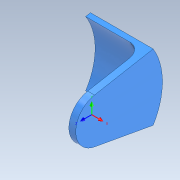
# Autodesk Inventor part: thigh_connector
Saved by Autodesk Inventor 2020 (Build 240168000, 168)
## iProperties
Created: 2021-03-27
Part Number: thigh_connector
Material: Generic
Document SubType Name: Modeling
Designer: DELL
Density: 1 g/cm^3
Appearance: Cyan
Author: DELL
Autodesk Inventor part; units mm, degrees
ref_plane "YZ Plane" through (0, 0, 0) normal (1, 0, 0) x (0, 1, 0)
ref_plane "XZ Plane" through (0, 0, 0) normal (0, 1, 0) x (-1, 0, 0)
ref_plane "XY Plane" through (0, 0, 0) normal (0, 0, 1) x (1, 0, 0)
sketch "Sketch1" plane through (0, 0, 0) normal (1, 0, 0) x (0, 1, 0)
  circle A0 centre (0, 0) radius 20
  line L0 (-19.68, 3.5636) -> (-29, -47.9062)
  line L1 (19.68, 3.5636) -> (29, -47.9062)
  line L2 (11.5, 0) -> (-11.5, 0) construction
  line L3 (0, -48.5721) -> (0, 48.5721) construction
  arc A1 (-28.2326, -43.6683) -> (28.2326, -43.6683) centre (0, 0) ccw
  arc A2 (-29, -47.9062) -> (29, -47.9062) centre (0, 0) ccw
  point P0 (0, -56)
  point P1 (0, 0)
  dimension "d0" = 40
  dimension "d8" = 104
  dimension "d9" = 112
  dimension "d10" = 58
  constraints: 8 end point, 7 point on circle, 5 coincident, 5 midpoint, 3 centre point, 2 point on line, 2 symmetric about line, 2 tangent, 1 horizontal, 1 vertical, 1 other
  measures "d0" diameter of A0
  measures "d8" diameter of A1
  measures "d9" diameter of A2
  measures "d10" distance of L1.end L0.end
extrude "Extrusion1" add sketch "Sketch1" along normal blind 6
extrude "Extrusion2" add sketch "Sketch1" against normal blind 49 contours L1 A2 L0 A1
fillet "Fillet1" radius 10 1 edges at (0, 0, -52)
body "Solid1"
